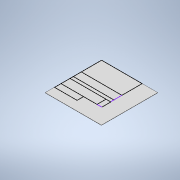
# Autodesk Inventor part: Part1
Saved by Autodesk Inventor 2022 (Build 260153000, 153)
## iProperties
Created: 2023-01-13
Part Number: Part1
Material: 一般
Document SubType Name: Modeling
Designer: tdn82
Density: 1 g/cm^3
Appearance: 既定
Author: tdn82
Autodesk Inventor part; units mm, degrees
ref_plane "YZ Plane" through (0, 0, 0) normal (1, 0, 0) x (0, 1, 0)
ref_plane "XZ Plane" through (0, 0, 0) normal (0, 1, 0) x (-1, 0, 0)
ref_plane "XY Plane" through (0, 0, 0) normal (0, 0, 1) x (1, 0, 0)
sketch "スケッチ1" plane through (0, 0, 0) normal (0, 1, 0) x (-1, 0, 0)
  line L0 (0, 0) -> (-500, 0)
  line L1 (-500, 0) -> (-500, -500)
  line L2 (-500, -500) -> (0, -500)
  line L3 (0, -500) -> (0, 0)
  dimension "d0" = 500
  dimension "d1" = 500
  constraints: 8 end point, 2 parallel, 1 horizontal, 1 perpendicular
  measures "d0" distance of L1.end L2.end
  measures "d1" distance of L0.end L1.end
extrude "押し出し1" add sketch "スケッチ1" along normal blind 2
sketch "スケッチ2" plane through (0, 2, 0) normal (0, 1, 0) x (1, 0, 0)
  line L0 (0, 500) -> (360, 500)
  line L1 (360, 500) -> (360, 320)
  line L2 (360, 320) -> (0, 320)
  line L3 (0, 320) -> (0, 500)
  line L4 (0, 320) -> (360, 320)
  line L5 (360, 320) -> (360, 249)
  line L6 (360, 249) -> (0, 249)
  line L7 (0, 249) -> (0, 320)
  line L8 (0, 249) -> (360, 249)
  line L9 (360, 249) -> (360, 220)
  line L10 (360, 220) -> (0, 220)
  line L11 (0, 220) -> (0, 249)
  line L12 (0, 220) -> (319.5, 220)
  line L13 (319.5, 220) -> (319.5, 140)
  line L14 (319.5, 140) -> (0, 140)
  line L15 (0, 140) -> (0, 220)
  line L16 (319.5, 220) -> (362, 220)
  line L17 (362, 220) -> (362, 140)
  line L18 (362, 140) -> (319.5, 140)
  line L19 (319.5, 140) -> (319.5, 220)
  line L20 (0, 140) -> (200, 140)
  line L21 (200, 140) -> (200, 82.5)
  line L22 (200, 82.5) -> (0, 82.5)
  line L23 (0, 82.5) -> (0, 140)
  dimension "d4" = 180
  dimension "d5" = 360
  dimension "d6" = 71
  dimension "d7" = 29
  dimension "d8" = 80
  dimension "d9" = 319.5
  dimension "d10" = 42.5
  dimension "d11" = 200
  dimension "d12" = 57.5
  constraints: 48 end point, 12 parallel, 6 horizontal, 6 perpendicular, 1 point on line
  measures "d4" distance of L0.end L1.end
  measures "d5" distance of L1.end L2.end
  measures "d6" distance of L4.end L5.end
  measures "d7" distance of L8.end L9.end
  measures "d8" distance of L12.end L13.end
  measures "d9" distance of L13.end L14.end
  measures "d10" distance between parallel lines of L17 L19
  measures "d11" distance of L21.end L22.end
  measures "d12" distance of L20.end L21.end
